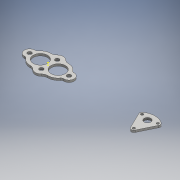
# Autodesk Inventor part: 240412_sketch
Saved by Autodesk Inventor 2016 (Build 200138000, 138)
## iProperties
Created: 2024-04-12
Part Number: 240412_sketch
Material: 일반
Document SubType Name: Modeling
Designer: pc
Density: 1 g/cm^3
Appearance: 기본값
Author: pc
Autodesk Inventor part; units mm, degrees
ref_plane "YZ Plane" through (0, 0, 0) normal (1, 0, 0) x (0, 1, 0)
ref_plane "XZ Plane" through (0, 0, 0) normal (0, 1, 0) x (-1, 0, 0)
ref_plane "XY Plane" through (0, 0, 0) normal (0, 0, 1) x (1, 0, 0)
sketch "스케치1" plane through (0, 0, 0) normal (0, 0, 1) x (1, 0, 0)
  circle A0 centre (43, 6.2877) radius 34.5
  circle A1 centre (-43, 6.2877) radius 34.5
  line L0 (-163.8708, 6.2877) -> (265.4786, 6.2877)
  circle A2 centre (95, 6.2877) radius 9.5
  circle A3 centre (-95, 6.2877) radius 9.5
  arc A4 (-93.5122, 31.2434) -> (-93.5122, -18.668) centre (-95, 6.2877) ccw
  arc A5 (93.5122, -18.668) -> (93.5122, 31.2434) centre (95, 6.2877) ccw
  line L1 (0, 109.3123) -> (0, -138.0954) construction
  arc A6 (-83.1597, -23.4981) -> (-93.5122, -18.668) centre (-92.7981, -30.6467) ccw
  arc A7 (93.5122, -18.668) -> (83.1597, -23.4981) centre (92.7981, -30.6467) ccw
  arc A8 (20.6273, 64.8842) -> (41.8953, 56.2755) centre (41.2545, 85.2684) ccw
  circle A9 centre (0, 44.5) radius 9.5
  circle A10 centre (0, -31.9246) radius 9.5
  arc A11 (-41.8953, 56.2755) -> (-20.6273, 64.8842) centre (-41.2545, 85.2684) ccw
  arc A12 (41.8953, -43.7001) -> (20.6273, -52.3088) centre (41.2545, -72.693) ccw
  arc A13 (-20.6273, -52.3088) -> (-41.8953, -43.7001) centre (-41.2545, -72.693) ccw
  arc A14 (83.1597, 36.0735) -> (93.5122, 31.2434) centre (92.7981, 43.2221) ccw
  arc A15 (-93.5122, 31.2434) -> (-83.1597, 36.0735) centre (-92.7981, 43.2221) ccw
  arc A16 (20.6273, 64.8842) -> (-20.6273, 64.8842) centre (0, 44.5) ccw
  arc A17 (-41.8953, 56.2755) -> (-83.1597, 36.0735) centre (-43, 6.2877) ccw
  arc A18 (-83.1597, -23.4981) -> (-41.8953, -43.7001) centre (-43, 6.2877) ccw
  arc A19 (83.1597, 36.0735) -> (41.8953, 56.2755) centre (43, 6.2877) ccw
  arc A20 (41.8953, -43.7001) -> (83.1597, -23.4981) centre (43, 6.2877) ccw
  arc A21 (-20.6273, -52.3088) -> (20.6273, -52.3088) centre (0, -31.9246) ccw
  point P0 (0, 0)
  point P1 (-42.3827, -0.6468)
  dimension "d0" = 69
  dimension "d1" = 69
  dimension "d5" = 19
  dimension "d8" = 19
  dimension "d9" = 95
  dimension "d11" = 95
  dimension "d15" = 50
  dimension "d16" = 50
  dimension "d19" = 43
  dimension "d20" = 43
  dimension "d25" = 24
  dimension "d26" = 24
  dimension "d27" = 58
  dimension "d28" = 19
  dimension "d30" = 44.5
  dimension "d34" = 58
  dimension "d35" = 58
  dimension "d36" = 58
  dimension "d37" = 24
  dimension "d38" = 24
  constraints: 32 point on circle, 22 centre point, 6 coincident, 5 point on line, 4 end point, 4 tangent, 2 horizontal, 2 symmetric about line, 2 vertical, 1 other
  measures "d0" diameter of A0
  measures "d1" diameter of A1
  measures "d5" diameter of A2
  measures "d8" diameter of A3
  measures "d9" horizontal distance of point (0, 0) A3.centre
  measures "d11" horizontal distance of point (0, 0) A2.centre
  measures "d15" diameter of A4
  measures "d16" diameter of A5
  measures "d19" horizontal distance of point (0, 0) A1.centre
  measures "d20" horizontal distance of point (0, 0) A0.centre
  measures "d25" diameter of A6
  measures "d26" diameter of A7
  measures "d27" diameter of A8
  measures "d28" diameter of A9
  measures "d30" distance of point (0, 0) A9.centre
  measures "d34" diameter of A11
  measures "d35" diameter of A12
  measures "d36" diameter of A13
  measures "d37" diameter of A14
  measures "d38" diameter of A15
extrude "돌출1" add sketch "스케치1" along normal blind 10 contours L0 A2 A5 A7 A20 A12 A21 A13 A18 A6 A4 A3 A1 A0 | A0 L0 A1 A3 A4 A15 A17 A11 A16 A8 A19 A14 A5 A2
sketch "스케치2" plane through (0, 0, 10) normal (0, 0, 1) x (1, 0, 0)
  point P0 (0, 0)
sketch "스케치3" plane through (0, 0, 10) normal (0, 0, 1) x (1, 0, 0)
  point P0 (0, 0)
sketch "스케치4" plane through (0, 0, 10) normal (0, 0, 1) x (1, 0, 0)
  line L0 (479.7309, 137.7571) -> (479.7309, -142.8376)
  line L1 (343.2747, -0.004) -> (642.8719, -0.004)
  circle A0 centre (479.7309, -0.004) radius 16
  circle A1 centre (479.7309, -66.004) radius 6
  circle A2 centre (517.7309, 11.996) radius 6
  circle A3 centre (441.7309, 11.996) radius 6
  arc A4 (468.6161, -70.5273) -> (490.7063, -70.8558) centre (479.7309, -66.004) ccw
  arc A5 (527.5635, 5.1171) -> (524.8559, 21.6518) centre (517.7309, 11.996) ccw
  arc A6 (434.6059, 21.6518) -> (430.9447, 6.737) centre (441.7309, 11.996) ccw
  line L2 (469.3219, -71.975) -> (430.9447, 6.737)
  line L3 (490.7063, -70.8558) -> (527.5635, 5.1171)
  arc A7 (524.8559, 21.6518) -> (434.6059, 21.6518) centre (479.7309, -39.5016) ccw
  point P0 (0, 0)
  dimension "d41" = 32
  dimension "d42" = 12
  dimension "d43" = 66
  dimension "d44" = 12
  dimension "d45" = 38
  dimension "d46" = 12
  dimension "d47" = 24
  dimension "d48" = 24
  dimension "d49" = 24
  dimension "d50" = 152
  constraints: 9 point on circle, 8 centre point, 8 end point, 5 point on line, 3 coincident, 2 tangent, 1 horizontal, 1 symmetric about line, 1 vertical, 1 other
  measures "d41" diameter of A0
  measures "d42" diameter of A1
  measures "d43" distance of A1.centre A0.centre
  measures "d44" diameter of A2
  measures "d45" horizontal distance of A2.centre A0.centre
  measures "d46" vertical distance of A2.centre A0.centre
  measures "d47" diameter of A4
  measures "d48" diameter of A5
  measures "d49" diameter of A6
  measures "d50" diameter of A7
extrude "돌출2" add sketch "스케치4" along normal blind 10 contours A7 A5 L3 L1 A0 L0 | L0 A0 L1 L2 A6 A7 | L1 L3 A4 L0 A1 A0 | A0 L0 A1 A4 L2 L1
sketch "스케치5" plane through (0, 0, 20) normal (0, 0, 1) x (1, 0, 0)
  point P0 (0, 0)
